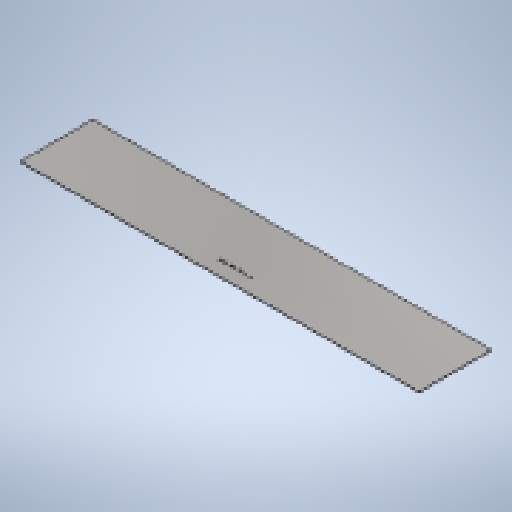
# Autodesk Inventor part: MSC 702 face 3
Saved by Autodesk Inventor 2025 (Build 290162010, 162A)
## iProperties
Created: 2024-06-16
Part Number: MSC 702 face 3
Material: Stainless Steel
Document SubType Name: Sheet Metal
Designer: admin
Density: 8 g/cm^3
Sheet Metal Rule: AISI304 2mm Die16
Appearance: Semi-Polished
Stock Number: МОО 702 морда 3
Author: admin
Autodesk Inventor part; units mm, degrees
ref_plane "YZ Plane" through (0, 0, 0) normal (1, 0, 0) x (0, 1, 0)
ref_plane "XZ Plane" through (0, 0, 0) normal (0, 1, 0) x (-1, 0, 0)
ref_plane "XY Plane" through (0, 0, 0) normal (0, 0, 1) x (1, 0, 0)
sketch "Sketch1" plane through (0, 0, 0) normal (0, 0, 1) x (1, 0, 0)
  line L0 (-734.0742, 0) -> (734.0742, 0)
  line L1 (734.0742, 0) -> (734.0742, -267.044)
  line L2 (734.0742, -267.044) -> (-734.0742, -267.044)
  line L3 (-734.0742, -267.044) -> (-734.0742, 0)
  point P0 (0, 0)
  point P1 (0, 0)
  dimension "d0" = 1468.1483
  dimension "d1" = 267.044
  measures "d0" distance of L1.end L2.end
  measures "d1" distance of L0.end L1.end
extrude "Plate1" add sketch "Sketch1" along normal blind 2
sketch "Sketch2" plane through (0, 0, 2) normal (0, 0, 1) x (1, 0, 0)
  line L0 (-55, -217.044) -> (-55, -205.044) construction
  line L1 (-55, -205.044) -> (55, -205.044) construction
  line L2 (55, -205.044) -> (55, -217.044) construction
  line L3 (55, -217.044) -> (-55, -217.044) construction
  line L4 (734.0742, -267.044) -> (-734.0742, -267.044) projected
  point P0 (0, 0)
  point P1 (0, -217.044)
  point P2 (0, -267.044)
  dimension "d3" = 12
  dimension "d4" = 110
  dimension "d5" = 50
  constraints: 2 midpoint, 1 vertical alignment, 2 other
  measures "d3" distance of L1.end L2.end
  measures "d4" distance between parallel lines of L0 L2
  measures "d5" distance between parallel lines of L4 L3
mark "Mark1"
equation "\"d2\" = Thickness"
equation "\"BendReliefWidth\" = Thickness"
equation "\"BendReliefDepth\" = 0.5 * Thickness"
equation "\"CornerReliefSize\" = 4 * Thickness"
equation "\"MinimumRemnant\" = 2 * Thickness"
equation "\"TransitionRadius\" = BendRadius"
equation "\"JacobiRadiusSize\" = BendRadius"
equation "\"GapSize\" = Thickness"
equation "\"Thickness\" = 2"
equation "\"BendRadius\" = 2.75"
body "Solid1"
